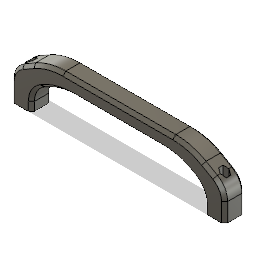
Enclosure v3 v8 (Autodesk Fusion 360 archive; units mm, degrees)
design "Handle"
Autodesk Fusion 360 part; units mm, degrees
sketch "Sketch1" plane through (0, 0, 0) normal (0, 0, 1) x (1, 0, 0)
  line L0 (0, 0) -> (0, 30)
  line L1 (35, 50) -> (175, 50)
  line L2 (105, 61.1727) -> (105, -24.9147) construction
  line L3 (20, 20) -> (45, 35)
  line L4 (45, 35) -> (165, 35)
  line L5 (165, 35) -> (190, 20)
  line L6 (210, 30) -> (210, 0)
  line L7 (0, 0) -> (20, 0)
  line L8 (20, 0) -> (20, 20)
  line L9 (210, 0) -> (190, 0)
  line L10 (190, 0) -> (190, 20)
  line L11 (35, 50) -> (0, 30)
  line L12 (175, 50) -> (210, 30)
  dimension "d1" = 210
  dimension "d5" = 140
  dimension "d7" = 15
  dimension "d14" = 50
  dimension "d16" = 20
  dimension "d18" = 20
  dimension "d24" = 120
  dimension "d37" = 30
  dimension "d38" = 20
  dimension "d39" = 20
  constraint coincident L0.start L7.start
  constraint perpendicular L0 L1
  constraint vertical L2
  constraint symmetric L0.start L6.end L2
  constraint symmetric L0.end L6.start L2
  constraint horizontal L4
  constraint symmetric L2 L3.end L4.end
  constraint perpendicular L0 L7
  constraint perpendicular L7 L8
  constraint perpendicular L6 L9
  constraint perpendicular L9 L10
  constraint symmetric L1.start L1.end L2
  measures "d1" distance of L0.start L6.end
  measures "d5" distance of L1.start L1.end
  measures "d7" distance of L1 L4
  measures "d14" distance of L0.start L1
  measures "d16" distance of L7.end L3.start
  measures "d18" distance of L9.end L5.end
  measures "d24" distance of L3.end L4.end
  measures "d37" distance of L0.start L0.end
  measures "d38" distance of L0.start L7.end
  measures "d39" distance of L6.end L9.end
extrude "Extrude1" add sketch "Sketch1" along normal blind 20
fillet "Fillet1" radius 20 4 edges at (20, 20, 10) (190, 20, 10) (0, 30, 10) (210, 30, 10)
fillet "Fillet1" radius 60 4 edges at (45, 35, 10) (165, 35, 10) (35, 50, 10) (175, 50, 10)
chamfer "Chamfer1" distance 3 angle 45 36 edges at (45.603, 32.8229, 20) (30.2297, 26.1378, 20) (22.596, 18.5302, 20) (20, 4.3381, 20) (190, 4.3381, 20) (187.404, 18.5302, 20) (179.7703, 26.1378, 20) (164.397, 32.8229, 20) (105, 35, 20) (105, 50, 20) (35.5338, 47.99, 20) (15.6214, 38.9265, 20) (2.7018, 28.4321, 20) (0, 9.1968, 20) (210, 9.1968, 20) (207.2982, 28.4321, 20) (194.3786, 38.9265, 20) (174.4662, 47.99, 20) (105, 50, 0) (174.4662, 47.99, 0) (194.3786, 38.9265, 0) (207.2982, 28.4321, 0) (210, 9.1968, 0) (0, 9.1968, 0) (2.7018, 28.4321, 0) (15.6214, 38.9265, 0) (35.5338, 47.99, 0) (105, 35, 0) (164.397, 32.8229, 0) (179.7703, 26.1378, 0) (187.404, 18.5302, 0) (190, 4.3381, 0) (20, 4.3381, 0) (22.596, 18.5302, 0) (30.2297, 26.1378, 0) (45.603, 32.8229, 0)
sketch "Sketch2" plane through (0, 0, 0) normal (0, 1, 0) x (1, 0, 0)
  line L0 (3, -20) -> (17, -20) construction
  line L1 (3, 0) -> (17, 0) construction
  line L2 (193, -20) -> (207, -20) construction
  line L3 (207, 0) -> (193, 0) construction
  line L4 (10, -20) -> (10, 0) construction
  line L5 (200, -20) -> (200, 0) construction
  circle A0 centre (10, -10) radius 2.25
  circle A1 centre (200, -10) radius 2.25
  line L6 (6.25, -12.1651) -> (10, -14.3301)
  line L7 (10, -14.3301) -> (13.75, -12.1651)
  line L8 (13.75, -12.1651) -> (13.75, -7.8349)
  line L9 (13.75, -7.8349) -> (10, -5.6699)
  line L10 (10, -5.6699) -> (6.25, -7.8349)
  line L11 (6.25, -7.8349) -> (6.25, -12.1651)
  line L12 (200, -5.6699) -> (196.25, -7.8349)
  line L13 (196.25, -7.8349) -> (196.25, -12.1651)
  line L14 (196.25, -12.1651) -> (200, -14.3301)
  line L15 (200, -14.3301) -> (203.75, -12.1651)
  line L16 (203.75, -12.1651) -> (203.75, -7.8349)
  line L17 (203.75, -7.8349) -> (200, -5.6699)
  point P0 (10, -10)
  point P1 (200, -10)
  dimension "d19" = 4.5
  dimension "d20" = 4.5
  dimension "d23" = 190
  dimension "d40" = 7.5
  dimension "d41" = 7.5
  constraint midpoint L0 L4.start
  constraint midpoint L1 L4.end
  constraint midpoint L2 L5.start
  constraint midpoint L3 L5.end
  constraint midpoint L4 P0
  constraint midpoint L5 P1
  constraint coincident P0 A0.centre
  constraint vertical L11
  constraint coincident P1 A1.centre
  constraint vertical L16
  measures "d19" diameter of A0
  measures "d20" diameter of A1
  measures "d23" distance of P0 P1
  measures "d40" distance of L8 L11
  measures "d41" distance of L13 L16
extrude "Extrude2" cut sketch "Sketch2" along normal blind 100 contours A0 | A1
extrude "Extrude3" cut sketch "Sketch2" along normal blind 50 from surface at 10 contours A1 | L6 L7 L8 L9 L10 L11 | L12 L13 L14 L15 L16 L17
equation "d18 = d16"
